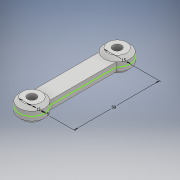
# Autodesk Inventor part: Деталь2_б
Saved by Autodesk Inventor 2018 (Build 220112000, 112)
## iProperties
Created: 2018-11-12
Part Number: Деталь2_б
Material: Типовые
Document SubType Name: Modeling
Designer: Lev
Density: 1 g/cm^3
Appearance: По умолчанию
Author: Lev
Autodesk Inventor part; units mm, degrees
ref_plane "YZ Plane" through (0, 0, 0) normal (1, 0, 0) x (0, 1, 0)
ref_plane "XZ Plane" through (0, 0, 0) normal (0, 1, 0) x (-1, 0, 0)
ref_plane "XY Plane" through (0, 0, 0) normal (0, 0, 1) x (1, 0, 0)
sketch "Эскиз1" plane through (0, 0, 0) normal (0, 0, 1) x (1, 0, 0)
  circle A0 centre (0, 25) radius 7.5
  circle A1 centre (0, -25) radius 7.5
  circle A2 centre (0, -25) radius 2.5
  circle A3 centre (0, 25) radius 2.5
  line L0 (-5, 19.4098) -> (-5, -19.4098)
  line L1 (5, 19.4098) -> (5, -19.4098)
  point P0 (0, 0)
  point P1 (-5, 0)
  dimension "d2" = 15
  dimension "d3" = 15
  dimension "d4" = 5
  dimension "d12" = 50
  constraints: 4 centre point, 4 end point, 4 point on circle, 2 coincident, 1 horizontal alignment, 1 vertical alignment
  measures "d2" diameter of A0
  measures "d3" diameter of A1
  measures "d4" diameter of A2
  measures "d12" distance of A1.centre A0.centre
extrude "Выдавливание1" add sketch "Эскиз1" along normal mid plane 5 contours A0 L1 A1 L0
extrude "Выдавливание2" add sketch "Эскиз1" along normal mid plane 9 contours A0 | A1
chamfer "Фаска1" distance 2 angle 45 4 edges at (5, 30.5902, 4.5) (5, 30.5902, -4.5) (-5, -30.5902, 4.5) (-5, -30.5902, -4.5)
